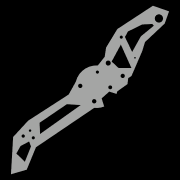
# Autodesk Inventor part: UpperLeg
Saved by Autodesk Inventor 2020 (Build 240168000, 168)
## iProperties
Created: 2020-05-08
Part Number: UpperLeg
Material: Generic
Document SubType Name: Sheet Metal
Designer: valer
Density: 1 g/cm^3
Sheet Metal Rule: Default
Appearance: Default
Author: valer
Autodesk Inventor part; units mm, degrees
ref_plane "YZ Plane" through (0, 0, 0) normal (1, 0, 0) x (0, 1, 0)
ref_plane "XZ Plane" through (0, 0, 0) normal (0, 1, 0) x (-1, 0, 0)
ref_plane "XY Plane" through (0, 0, 0) normal (0, 0, 1) x (1, 0, 0)
sketch "Sketch1" plane through (0, 0, 0) normal (0, 0, 1) x (1, 0, 0)
  circle A0 centre (274.6375, 230.1875) radius 63.7776
  line L0 (337.2363, 403.1568) -> (443.981, 473.0492)
  line L1 (492.3212, 456.2573) -> (443.981, 473.0492)
  line L2 (492.2503, 456.2819) -> (479.284, 419.7573)
  line L3 (24.5719, 79.2848) -> (18.0689, -32.4356)
  line L4 (72.5364, 65.9043) -> (46.6491, 52.2142)
  line L5 (46.6491, 52.2142) -> (34.0412, 29.6597)
  line L6 (255.7975, 256.9468) -> (289.4332, 262.5767)
  line L7 (246.0625, 230.9446) -> (304.4287, 240.5522)
  line L8 (255.7975, 206.8518) -> (295.5251, 214.7787)
  circle A1 centre (461.9625, 434.975) radius 12.6457
  line L9 (407.8074, 381.2182) -> (381.6527, 334.3265)
  line L10 (369.0301, 396.0805) -> (359.9951, 379.3949)
  line L11 (347.7694, 356.8169) -> (320.0535, 305.6318)
  line L12 (379.495, 286.3527) -> (340.7579, 286.3527)
  line L13 (346.9208, 358.7018) -> (379.495, 286.3527)
  line L14 (442.324, 418.5388) -> (446.7794, 413.0787)
  line L15 (369.0301, 396.0805) -> (411.8405, 416.9757)
  line L16 (303.4865, 347.6193) -> (299.4344, 320.1261)
  line L17 (337.2363, 403.1568) -> (303.4865, 347.6193)
  line L18 (320.0535, 305.6318) -> (340.7579, 286.3527)
  line L19 (312.9368, 215.5598) -> (334.6972, 208.7305)
  line L20 (289.9762, 195.2062) -> (297.6262, 170.6972)
  line L21 (289.9762, 195.2062) -> (312.9368, 215.5598)
  line L22 (411.9572, 337.3855) -> (379.6015, 262.4018)
  line L23 (420.064, 364.1295) -> (411.9572, 337.3855)
  line L24 (359.9951, 379.3949) -> (381.6527, 334.3265)
  line L25 (212.6195, 245.0651) -> (191.178, 206.6512)
  line L26 (185.7375, 177.8) -> (227.516, 175.1568)
  line L27 (227.516, 175.1568) -> (105.2533, 88.1864)
  line L28 (336.8404, 216.103) -> (367.5606, 238.0391)
  line L29 (311.5134, 196.3392) -> (293.439, 184.1121)
  line L30 (267.8125, 166.7762) -> (92.8667, 48.4277)
  line L31 (420.064, 364.1295) -> (479.284, 419.7573)
  line L32 (411.8405, 416.9757) -> (442.324, 418.5388)
  line L33 (407.8074, 381.2182) -> (446.7794, 413.0787)
  line L34 (69.5552, 128.1105) -> (191.178, 206.6512)
  line L35 (18.0689, -32.4356) -> (65.2214, -18.7927)
  line L36 (34.0412, 29.6597) -> (59.7385, 4.8239)
  line L37 (185.7375, 177.8) -> (103.7911, 122.0067)
  line L38 (78.1426, 50.9035) -> (59.7385, 4.8239)
  line L39 (48.6888, -22.8421) -> (48.0458, -23.7622)
  line L40 (72.5364, 65.9043) -> (78.1426, 50.9035)
  line L41 (65.2214, -18.7927) -> (92.8667, 48.4277)
  line L42 (103.7911, 122.0067) -> (105.2533, 88.1864)
  line L43 (69.5552, 128.1105) -> (24.5719, 79.2848)
  circle A2 centre (75.3395, 98.5167) radius 3.8669
  circle A3 centre (84.9883, 76.8485) radius 4.9522
  circle A4 centre (54.6855, 82.1395) radius 5.1805
  circle A5 centre (315.8668, 228.3626) radius 6.0269
  circle A6 centre (277.3871, 274.0573) radius 4.9522
  circle A7 centre (225.9204, 232.6915) radius 6.6995
  circle A8 centre (267.7671, 186.5158) radius 6.8363
  circle A9 centre (353.305, 262.674) radius 6.644
  circle A10 centre (349.0556, 378.9146) radius 4.9052
  circle A11 centre (390.0304, 316.8931) radius 2.5174
  circle A12 centre (309.84, 301.1277) radius 7.816
  line L44 (369.7695, 256.03) -> (379.6015, 262.4018)
  line L45 (369.7695, 256.03) -> (367.5606, 238.0391)
  line L46 (299.4344, 320.1261) -> (278.7261, 293.8339)
  line L47 (232.2646, 234.8443) -> (231.9064, 234.3894)
extrude "Plate1" add sketch "Sketch1" along normal blind 3.048 contours A0 L19 L21 L20 | A0 L46 L16 L17 L0 L1 L2 L31 L23 L22 L44 L45 L28 | A0 L30 L41 L35 L3 L43 L34 L25 picked at (259.3337, 231.7117)
equation "\"d0\" = Thickness"
equation "\"BendRadius\" = Thickness"
equation "\"BendReliefWidth\" = Thickness"
equation "\"BendReliefDepth\" = 0.5 * Thickness"
equation "\"CornerReliefSize\" = 4 * Thickness"
equation "\"MinimumRemnant\" = 2 * Thickness"
equation "\"TransitionRadius\" = BendRadius"
equation "\"JacobiRadiusSize\" = BendRadius"
equation "\"GapSize\" = Thickness"
equation "\"Thickness\" = 3.048"
body "Solid1"
